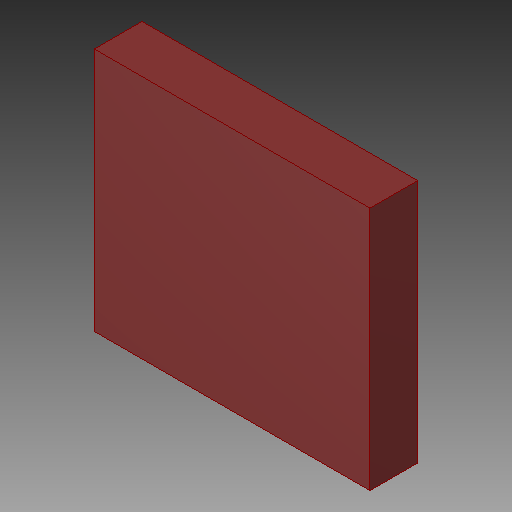
# Autodesk Inventor part: RGBLED_CA-5MM
Saved by Autodesk Inventor 2019 (Build 230136000, 136)
## iProperties
Created: 2019-10-02
Part Number: RGBLED_CA-5MM
Material: Generic
Document SubType Name: Modeling
Designer: rybit
Density: 1 g/cm^3
Appearance: LED5MMRGB, RGBLED_CA-5MM
Author: rybit
Autodesk Inventor part; units mm, degrees
ref_plane "YZ Plane" through (0, 0, 0) normal (1, 0, 0) x (0, 1, 0)
ref_plane "XZ Plane" through (0, 0, 0) normal (0, 1, 0) x (-1, 0, 0)
ref_plane "XY Plane" through (0, 0, 0) normal (0, 0, 1) x (1, 0, 0)
sketch "LED5MMRGB, RGBLED_CA-5MM_21" plane through (0, 0, 0) normal (0, 0, 1) x (1, 0, 0)
  line L0 (-2.6035, 2.5635) -> (3.175, 2.5635)
  line L1 (3.175, 2.5635) -> (3.175, -2.5635)
  line L2 (3.175, -2.5635) -> (-2.6035, -2.5635)
  line L3 (-2.6035, -2.5635) -> (-2.6035, 2.5635)
  constraints: 8 end point
extrude "Extrusion1" add sketch "LED5MMRGB, RGBLED_CA-5MM_21" along normal blind 1
body "Solid1"
